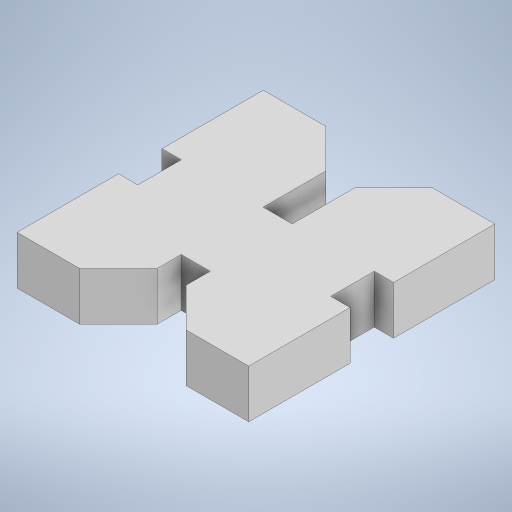
# Autodesk Inventor part: Vblock
Saved by Autodesk Inventor 2024 (Build 280153000, 153)
## iProperties
Created: 2024-02-05
Part Number: Vblock
Material: Generisch
Document SubType Name: Modeling
Designer: ffogue
Density: 1 g/cm^3
Appearance: Vorgabe
Author: ffogue
Autodesk Inventor part; units mm, degrees
ref_plane "YZ Plane" through (0, 0, 0) normal (1, 0, 0) x (0, 1, 0)
ref_plane "XZ Plane" through (0, 0, 0) normal (0, 1, 0) x (-1, 0, 0)
ref_plane "XY Plane" through (0, 0, 0) normal (0, 0, 1) x (1, 0, 0)
sketch "Skizze1" plane through (0, 0, 0) normal (0, 0, 1) x (1, 0, 0)
  line L0 (13, 0) -> (0, 0)
  line L1 (0, 0) -> (0, 21)
  line L2 (0, 21) -> (4, 21)
  line L3 (4, 21) -> (4, 30)
  line L4 (4, 30) -> (0, 30)
  line L5 (0, 30) -> (0, 51)
  line L6 (0, 51) -> (13, 51)
  line L7 (13, 51) -> (21, 43)
  line L8 (21, 43) -> (21, 30)
  line L9 (21, 30) -> (27, 30)
  line L10 (27, 30) -> (27, 43)
  line L11 (27, 43) -> (35, 51)
  line L12 (35, 51) -> (48, 51)
  line L13 (48, 51) -> (48, 30)
  line L14 (48, 30) -> (44, 30)
  line L15 (44, 30) -> (44, 21)
  line L16 (44, 21) -> (48, 21)
  line L17 (48, 21) -> (48, 0)
  line L18 (48, 0) -> (35, 0)
  line L19 (35, 0) -> (27, 8)
  line L20 (27, 8) -> (27, 13)
  line L21 (27, 13) -> (21, 13)
  line L22 (21, 13) -> (21, 8)
  line L23 (21, 8) -> (13, 0)
  point P0 (48, 40.5)
  point P1 (41.5, 51)
  dimension "d0" = 21
  dimension "d1" = 9
  dimension "d2" = 21
  dimension "d3" = 21
  dimension "d4" = 21
  dimension "d5" = 4
  dimension "d6" = 4
  dimension "d7" = 13
  dimension "d8" = 22
  dimension "d9" = 13
  dimension "d10" = 21
  dimension "d11" = 135
  dimension "d12" = 135
  dimension "d13" = 45
  dimension "d14" = 45
  constraints: 49 end point, 14 perpendicular, 6 point on line, 4 horizontal alignment, 2 collinear, 2 midpoint, 2 vertical alignment, 1 coincident, 1 horizontal, 1 parallel, 1 vertical
  measures "d0" distance between parallel lines of L0 L2
  measures "d1" distance between parallel lines of L2 L4
  measures "d2" distance of L4.end L5.end
  measures "d3" distance from line of L5.end L8
  measures "d4" distance from line of L12.end L10
  measures "d5" distance between parallel lines of L5 L3
  measures "d6" distance from line of point (48, 40.5) L15
  measures "d7" distance of L0.start L0.end
  measures "d8" distance of L18.end L0.start
  measures "d9" distance between parallel lines of L18 L21
  measures "d10" distance from line of point (41.5, 51) L9
  measures "d11" angle of L0 L23
  measures "d12" angle of L18 L19
  measures "d13" angle of L6 L7
  measures "d14" angle of L12 L11
extrude "Extrusion1" add sketch "Skizze1" against normal blind 10
equation "\"d2\" = d0"
equation "\"d4\" = d3"
equation "\"d6\" = d5"
equation "\"d10\" = d0"
equation "\"d14\" = d13"
